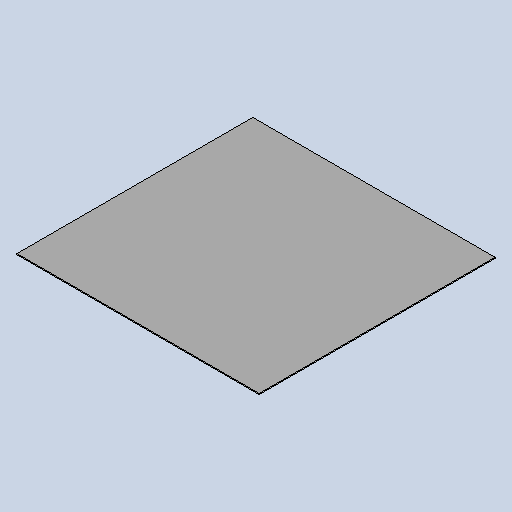
# Autodesk Inventor part: PNS waste water bin 02
Saved by Autodesk Inventor 2025.3 (Build 293356030, 356C)
## iProperties
Created: 2025-09-03
Part Number: PNS waste water bin 02
Material: Generic
Document SubType Name: Sheet Metal
Designer: admin
Density: 1 g/cm^3
Sheet Metal Rule: Default
Appearance: Default
Flat Pattern Width: 48 cm
Flat Pattern Length: 49.3 cm
Flat Pattern Area: 2366.4 cm^2
Sheet Metal Width: 480,000 mm
Sheet Metal Length: 493,000 mm
Sheet Metal Area: 236640,000 mm^2
Mass: 473.28 g
Surface Area: 4771.72 cm^2
Volume: 473.28 cm^3
Author: admin
Autodesk Inventor part; units mm, degrees
ref_plane "YZ Plane" through (0, 0, 0) normal (1, 0, 0) x (0, 1, 0)
ref_plane "XZ Plane" through (0, 0, 0) normal (0, 1, 0) x (-1, 0, 0)
ref_plane "XY Plane" through (0, 0, 0) normal (0, 0, 1) x (1, 0, 0)
sketch "Sketch1" plane through (0, 0, 0) normal (0, 0, 1) x (1, 0, 0)
  line L0 (285, 285) -> (-285, -285) construction
  line L1 (-246.5, -240) -> (246.5, -240)
  line L2 (246.5, -240) -> (246.5, 240)
  line L3 (246.5, 240) -> (-246.5, 240)
  line L4 (-246.5, 240) -> (-246.5, -240)
  line L5 (-246.5, -240) -> (246.5, 240) construction
  line L6 (246.5, -240) -> (-246.5, 240) construction
  point P0 (0, 0)
  dimension "d2" = 493
  dimension "d18" = 480
  measures "d2" distance of L3.end L2.end
  measures "d18" distance of L1.end L2.end
extrude "Plate1" add sketch "Sketch1" along normal blind 2
equation "\"d3\" = Thickness"
equation "\"BendRadius\" = Thickness"
equation "\"BendReliefWidth\" = Thickness"
equation "\"BendReliefDepth\" = 0.5 * Thickness"
equation "\"CornerReliefSize\" = 4 * Thickness"
equation "\"MinimumRemnant\" = 2 * Thickness"
equation "\"TransitionRadius\" = BendRadius"
equation "\"JacobiRadiusSize\" = BendRadius"
equation "\"GapSize\" = Thickness"
equation "\"Thickness\" = 2"
body "Solid1"
